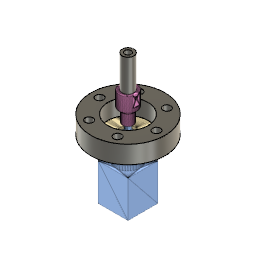
Zapfsäule (Autodesk Fusion 360 design; units mm, degrees)
Autodesk Fusion 360 part; units mm, degrees
sketch "Skizze1" plane through (0, 0, 0) normal (0, 0, 1) x (1, 0, 0)
  circle A0 centre (0, 0) radius 52
  dimension "d1" = 104
  constraint coincident A0.centre origin
  measures "d1" diameter of A0
extrude "Extrusion1" add sketch "Skizze1" along normal blind 25 makes body 1
sketch "Skizze2" plane through (0, 0, 0) normal (0, 0, 1) x (1, 0, 0)
  circle A0 centre (0, 0) radius 48
  dimension "d4" = 96
  constraint coincident A0.centre origin
  measures "d4" diameter of A0
extrude "Extrusion2" cut sketch "Skizze2" along normal blind 3 bodies 1
sketch "Skizze3" plane through (0, 0, 0) normal (0, 0, 1) x (1, 0, 0)
  circle A0 centre (0, 0) radius 28.25
  dimension "d7" = 56.5
  constraint coincident A0.centre origin
  measures "d7" diameter of A0
extrude "Extrusion3" cut sketch "Skizze3" along normal blind 25 bodies 1
sketch "Skizze4" plane through (0, 0, 0) normal (0, 0, 1) x (1, 0, 0)
  circle A0 centre (40, 0) radius 5.5
  circle A1 centre (20, 34.641) radius 5.5
  circle A2 centre (-20, 34.641) radius 5.5
  circle A3 centre (-40, 0) radius 5.5
  circle A4 centre (-20, -34.641) radius 5.5
  circle A5 centre (20, -34.641) radius 5.5
  dimension "d10" = 11
  dimension "d11" = 40
  dimension "d13" = 360
  measures "d10" diameter of A0
  measures "d11" distance of origin A0.centre
extrude "Extrusion4" cut sketch "Skizze4" along normal blind 25 bodies 1
sketch "Skizze5" plane through (0, 0, 0) normal (0, 0, 1) x (1, 0, 0)
  circle A0 centre (0, 0) radius 8.35
  dimension "d16" = 16.7
  constraint coincident A0.centre origin
  measures "d16" diameter of A0
extrude "Extrusion5" add sketch "Skizze5" along normal blind 41 and the other way blind -100 separate body makes body 2
sketch "Skizze6" plane through (0, 0, 0) normal (0, 0, 1) x (1, 0, 0)
  circle A0 centre (0, 0) radius 4.5
  dimension "d21" = 9
  constraint coincident A0.centre origin
  measures "d21" diameter of A0
extrude "Extrusion6" cut sketch "Skizze6" along normal blind 100 bodies 2
sketch "Skizze7" plane through (0, 0, 0) normal (0, 0, 1) x (1, 0, 0)
  line L0 (-13.6138, 1.5) -> (17.075, 1.5)
  line L1 (17.075, 1.5) -> (17.075, -1.5)
  line L2 (17.075, -1.5) -> (-13.6138, -1.5)
  line L3 (-13.6138, -1.5) -> (-13.6138, 1.5)
  line L4 (1.75, 0) -> (22.5, 0)
  dimension "d24" = 3
  constraint horizontal L0
  constraint vertical L1
  constraint horizontal L2
  constraint vertical L3
  constraint symmetric L0 L2 L4
  measures "d24" distance of L0.end L1.end
extrude "Extrusion7" cut sketch "Skizze7" along normal blind 50.5 bodies 2
other "Grundnetzelement1"
other "Grundnetzelement2"
other "Grundnetzelement3"
